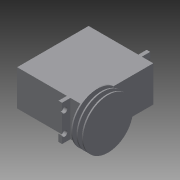
# Autodesk Inventor part: Whinch Servo
Saved by Autodesk Inventor 2014 SP1 (Build 180222100, 222)
## iProperties
Created: 2013-02-01
Part Number: Whinch Servo
Material: Generic
Document SubType Name: Modeling
Designer: Erik
Density: 1 g/cm^3
Appearance: Default
Author: Erik
Autodesk Inventor part; units mm, degrees
ref_plane "YZ Plane" through (0, 0, 0) normal (1, 0, 0) x (0, 1, 0)
ref_plane "XZ Plane" through (0, 0, 0) normal (0, 1, 0) x (-1, 0, 0)
ref_plane "XY Plane" through (0, 0, 0) normal (0, 0, 1) x (1, 0, 0)
sketch "Sketch1" plane through (0, 0, 0) normal (1, 0, 0) x (0, 1, 0)
  line L0 (0, 0) -> (60, 0)
  line L1 (60, 0) -> (60, 30)
  line L2 (60, 30) -> (0, 30)
  line L3 (0, 30) -> (0, 0)
  dimension "d0" = 60
  dimension "d2" = 30
  constraints: 8 end point, 2 parallel, 1 horizontal, 1 perpendicular
  measures "d0" distance of L1.end L2.end
  measures "d2" distance of L2.end L0.start
extrude "Extrusion1" add sketch "Sketch1" along normal blind 41.7
sketch "Sketch2" plane through (41.7, 0, 0) normal (1, 0, 0) x (0, 0, -1)
  line L0 (0, 0) -> (0, 60) projected
  line L1 (0, 60) -> (-30, 60) projected
  line L2 (-30, 60) -> (-30, 0) projected
  line L3 (-30, 0) -> (0, 0) projected
  line L4 (-30, 60) -> (0, 60)
  line L5 (0, 60) -> (0, 67)
  line L6 (-30, 67) -> (-30, 60)
  line L7 (-30, 0) -> (0, 0)
  line L8 (0, 0) -> (0, -7)
  line L9 (-30, -7) -> (-30, 0)
  arc A0 (-23.9717, 67) -> (-23.0283, 67) centre (-23.5, 64.8) ccw
  arc A1 (-6.9717, 67) -> (-6.0283, 67) centre (-6.5, 64.8) ccw
  arc A2 (-23.0283, -7) -> (-23.9717, -7) centre (-23.5, -4.8) ccw
  arc A3 (-6.0283, -7) -> (-6.9717, -7) centre (-6.5, -4.8) ccw
  line L10 (-23.9717, 67) -> (-30, 67)
  line L11 (0, 67) -> (-6.0283, 67)
  line L12 (-6.9717, 67) -> (-23.0283, 67)
  line L13 (-23.9717, -7) -> (-30, -7)
  line L14 (0, -7) -> (-6.0283, -7)
  line L15 (-6.9717, -7) -> (-23.0283, -7)
  dimension "d5" = 7
  dimension "d7" = 7
  dimension "d8" = 17
  dimension "d9" = 17
  dimension "d12" = 6.5
  dimension "d13" = 6.5
  dimension "d14" = 4.5
  dimension "d15" = 4.5
  dimension "d16" = 4.5
  dimension "d17" = 4.5
  constraints: 24 end point, 8 parallel, 8 point on circle, 4 centre point, 2 horizontal, 2 perpendicular
  measures "d5" distance of L7.end L8.end
  measures "d7" distance of L4.end L5.end
  measures "d8" distance of A3.centre A2.centre
  measures "d9" distance of A1.centre A0.centre
  measures "d12" distance from line of L8 A3.centre
  measures "d13" distance from line of L5 A1.centre
  measures "d14" diameter of A0
  measures "d15" diameter of A1
  measures "d16" diameter of A2
  measures "d17" diameter of A3
extrude "Extrusion2" add sketch "Sketch2" along normal blind 3
sketch "Sketch3" plane through (44.7, 0, 0) normal (1, 0, 0) x (0, 0, -1)
  line L0 (-30, 67) -> (-30, -7) projected
  line L1 (-30, 60) -> (0, 60)
  line L2 (0, 60) -> (0, 0)
  line L3 (0, 0) -> (-30, 0)
  line L4 (-30, 0) -> (-30, 60)
  dimension "d20" = 60
  constraints: 8 end point, 2 parallel, 1 horizontal, 1 perpendicular, 1 point on line
  measures "d20" distance between parallel lines of L1 L3
extrude "Extrusion3" add sketch "Sketch3" along normal blind 9.6
sketch "Sketch4" plane through (54.3, 0, 0) normal (1, 0, 0) x (0, 0, -1)
  line L0 (-30, 0) -> (0, 0) projected
  line L1 (0, 0) -> (0, 60) projected
  circle A0 centre (-15, 12) radius 2.5
  circle A1 centre (-15, 12) radius 21
  dimension "d24" = 5
  dimension "d25" = 15
  dimension "d26" = 12
  dimension "d27" = 42
  constraints: 2 centre point, 1 coincident
  measures "d24" diameter of A0
  measures "d25" distance from line of L1 A0.centre
  measures "d26" distance from line of L0 A0.centre
  measures "d27" diameter of A1
extrude "Extrusion4" add sketch "Sketch4" along normal blind 1 contours A0 | A1
sketch "Sketch5" plane through (55.3, 12, 15) normal (1, 0, 0) x (0, 0, -1)
  circle A0 centre (0, 0) radius 21 projected
  circle A1 centre (0, 0) radius 15
  point P0 (15, -12)
  dimension "d30" = 30
  constraints: 1 centre point, 1 coincident
  measures "d30" diameter of A1
extrude "Extrusion5" add sketch "Sketch5" along normal blind 3.5 contours A1
sketch "Sketch6" plane through (58.8, 12, 15) normal (1, 0, 0) x (0, 0, -1)
  circle A0 centre (0, 0) radius 15 projected
  circle A1 centre (0, 0) radius 21
  point P0 (15, -12)
  dimension "d33" = 42
  constraints: 1 centre point, 1 coincident
  measures "d33" diameter of A1
extrude "Extrusion6" add sketch "Sketch6" along normal blind 1 contours A0 | A1
sketch "Sketch7" plane through (59.8, 12, 15) normal (1, 0, 0) x (0, 0, -1)
  circle A0 centre (0, 0) radius 21 projected
  circle A1 centre (0, 0) radius 15
  point P0 (15, -12)
  dimension "d36" = 30
  constraints: 1 centre point, 1 coincident
  measures "d36" diameter of A1
extrude "Extrusion7" add sketch "Sketch7" along normal blind 3.5 contours A1
sketch "Sketch8" plane through (63.3, 12, 15) normal (1, 0, 0) x (0, 0, -1)
  circle A0 centre (0, 0) radius 15 projected
  circle A1 centre (0, 0) radius 21
  point P0 (15, -12)
  dimension "d39" = 42
  constraints: 1 centre point, 1 coincident
  measures "d39" diameter of A1
extrude "Extrusion8" add sketch "Sketch8" along normal blind 1 contours A0 | A1
body "Solid1"
